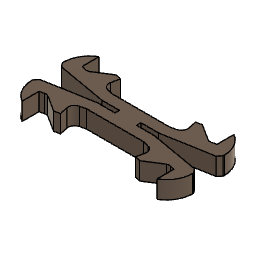
Track_Coupler (Autodesk Fusion 360 design; units mm, degrees)
Autodesk Fusion 360 part; units mm, degrees
sketch "Sketch1" plane through (0, 0, 0) normal (0, 0, 1) x (1, 0, 0)
  line L0 (-5, 0.3394) -> (-1.667, 0.3394)
  line L1 (-8, 2.6415) -> (-8, 4.0495)
  line L2 (-5, 4.2995) -> (-8, 4.2995)
  line L3 (-13, -3.75) -> (-13, -5.9)
  line L4 (-5, 3.75) -> (-13, -3.75) construction
  line L5 (11, -5.9) -> (11, -3.75)
  line L6 (-13, -3.75) -> (-21.1942, -3.75) construction
  line L7 (-5, -0.3394) -> (-11, -0.3394)
  line L8 (5, 0.3394) -> (2.3, 0.3394)
  line L9 (-13, 3.75) -> (-13, 5.9)
  line L10 (11, 5.9) -> (11, 3.3066)
  line L11 (-8, -5.75) -> (-8, -4.05)
  line L12 (-11, 5.9) -> (-11, 3.75)
  line L13 (-1.667, 0.3394) -> (-1.667, -0.3394)
  line L14 (-5, -4.05) -> (-5, -4.3)
  line L15 (13, -3.75) -> (5, -3.75)
  line L16 (13, 1.75) -> (5, 0.3394)
  line L17 (-13, -3.75) -> (-13, -1.75)
  line L18 (-1.667, -0.3394) -> (-5, -0.3394)
  line L19 (-13, -3.75) -> (-13, 3.75)
  line L20 (-13, 5.9) -> (-11, 5.9)
  line L21 (-13, -1.75) -> (-5, -0.3394)
  line L22 (-13, -3.75) -> (-5, -1.9764)
  line L23 (13, 3.75) -> (13, 5.9)
  line L24 (11, -3.75) -> (11, -3.3066)
  line L25 (-8, -4.3) -> (-8, -4.05)
  line L26 (13, -3.75) -> (5, -1.9764)
  line L27 (-13, 3.75) -> (-21.1942, 3.75) construction
  line L28 (13, 3.75) -> (5, 1.9764)
  line L29 (-11, -5.9) -> (-11, -3.3066)
  line L30 (13, -3.75) -> (13, -5.9)
  line L31 (-8, 4.0495) -> (-5, 4.0495)
  line L32 (-8, -4.05) -> (-8, -2.6415)
  line L33 (13, -3.75) -> (5, 3.75) construction
  line L34 (13, 3.75) -> (21.1942, 3.75) construction
  line L35 (-5, -4.05) -> (-5, -1.9764)
  line L36 (-11, 3.75) -> (-11, 3.3066)
  line L37 (13, 3.75) -> (13, -3.75)
  line L38 (-13, 3.75) -> (-5, -3.75) construction
  line L39 (-5, -0.3394) -> (-5, 0.3394)
  line L40 (-8, 4.2995) -> (-8, 4.0495)
  line L41 (13, -3.75) -> (13, -1.75)
  line L42 (-13, 3.75) -> (-13, 1.75)
  line L43 (13, 5.9) -> (11, 5.9)
  line L44 (-5, 1.9764) -> (-5, -1.9764)
  line L45 (-8, -4.05) -> (-5, -4.05)
  line L46 (5, -0.3394) -> (2.3, -0.3394)
  line L47 (-13, 3.75) -> (-5, 3.75)
  line L48 (5, 3.75) -> (13, 3.75)
  line L49 (-5, -4.3) -> (-8, -4.3)
  line L50 (2.3, 0.3394) -> (2.3, -0.3394)
  line L51 (-8, -4.05) -> (-5, -4.05)
  line L52 (13, -1.75) -> (5, -0.3394)
  line L53 (5, -3.75) -> (5, 3.75)
  line L54 (-13, 3.75) -> (-5, 1.9764)
  line L55 (13, 3.75) -> (13, 1.75)
  line L56 (13, 1.75) -> (21.1234, 1.75) construction
  line L57 (13, -5.9) -> (11, -5.9)
  line L58 (-13, -5.9) -> (-11, -5.9)
  line L59 (5, -3.75) -> (13, 3.75) construction
  line L60 (-8, 4.0495) -> (-5, 4.0495)
  line L61 (-5, -3.75) -> (-13, -3.75)
  line L62 (5, -1.9764) -> (5, 1.9764)
  line L63 (-13, 1.75) -> (-5, 0.3394)
  line L64 (-5, 4.0495) -> (-5, 1.9764)
  line L65 (-13, -1.75) -> (-21.1234, -1.75) construction
  line L66 (13, -3.75) -> (21.1942, -3.75) construction
  line L67 (-5, 4.0495) -> (-5, 4.2995)
  line L68 (0, -1.9764) -> (0, 1.9764)
  line L69 (5, 1.9764) -> (1.3, 1.9764)
  line L70 (0, 1.9764) -> (-5, 1.9764)
  line L71 (-5, -1.9764) -> (0, -1.9764)
  line L72 (1.3, -1.9764) -> (5, -1.9764)
  line L73 (1.3, 1.9764) -> (1.3, -1.9764)
  line L74 (-1.667, 0.3394) -> (-2.3, 0.3394)
  line L75 (-2.3, -0.3394) -> (-2.3, 0.3394)
  line L76 (-8, 4.2995) -> (-9.4644, 4.6242)
  line L77 (-9.4644, 4.6242) -> (-9.8148, 3.0439)
  line L78 (-8, 4.2995) -> (-5, 3.6344)
  line L79 (-9.4644, 4.6242) -> (-6.5356, 3.9749)
  line L80 (-6.5356, 3.9749) -> (-6.8859, 2.3945)
  line L81 (-9.4644, 4.6242) -> (-9.3238, 5.2588)
  line L82 (-6.5356, 3.9749) -> (-6.3949, 4.6095)
  line L83 (-9.3238, 5.2588) -> (-6.3949, 4.6095)
  point P0 (9, 0)
  point P1 (9, 0)
  point P2 (-9, 0)
  point P3 (-9, 0)
  dimension "d1" = 8
  dimension "d2" = 7.5
  dimension "d3" = 167.5
  dimension "d4" = 167.5
  dimension "d5" = 2
  dimension "d6" = 2
  dimension "d7" = 10
  dimension "d8" = 170
  dimension "d9" = 160
  dimension "d10" = 2.15
  dimension "d11" = 2
  dimension "d12" = 2.15
  dimension "d13" = 2
  dimension "d14" = 2.7
  dimension "d15" = 2.7
  dimension "d16" = 8
  dimension "d17" = 7.5
  dimension "d18" = 167.5
  dimension "d19" = 167.5
  dimension "d20" = 2
  dimension "d21" = 2
  dimension "d22" = 170
  dimension "d23" = 160
  dimension "d24" = 2.15
  dimension "d25" = 2
  dimension "d26" = 2.15
  dimension "d27" = 2
  dimension "d28" = 3.333
  dimension "d29" = 1.7
  dimension "d30" = 1.408
  dimension "d31" = 0.25
  dimension "d32" = 0.25
  dimension "d40" = 0.633
  dimension "d48" = 1.5
  dimension "d49" = 3
  dimension "d50" = 0.65
  dimension "d51" = 0.65
  constraint horizontal L15
  constraint perpendicular L15 L53
  constraint parallel L15 L48
  constraint parallel L37 L53
  constraint coincident P1 L33
  constraint coincident P1 L59
  constraint coincident P1 P0
  constraint horizontal L34
  constraint coincident L28.end L53
  constraint horizontal L66
  constraint coincident L26.end L53
  constraint perpendicular L48 L55
  constraint perpendicular L41 L66
  constraint horizontal L69
  constraint vertical L44
  constraint horizontal L71
  constraint vertical L62
  constraint horizontal L56
  constraint coincident L8.start L53
  constraint coincident L46.start L62
  constraint perpendicular L23 L48
  constraint perpendicular L23 L43
  constraint coincident L10.end L28
  constraint perpendicular L10 L43
  constraint perpendicular L15 L30
  constraint perpendicular L30 L57
  constraint coincident L5.end L15
  constraint perpendicular L5 L15
  constraint coincident L24.end L26
  constraint perpendicular L15 L24
  constraint perpendicular L8 L53
  constraint perpendicular L46 L53
  constraint parallel L47 L61
  constraint coincident P3 L38
  constraint coincident P3 L4
  constraint coincident P3 P2
  constraint perpendicular L17 L61
  constraint perpendicular L27 L42
  constraint perpendicular L3 L61
  constraint perpendicular L3 L58
  constraint coincident L29.end L22
  constraint perpendicular L29 L58
  constraint perpendicular L9 L47
  constraint perpendicular L9 L20
  constraint coincident L12.end L47
  constraint perpendicular L12 L47
  constraint coincident L36.end L54
  constraint perpendicular L36 L47
  constraint horizontal L0
  constraint vertical L13
  constraint horizontal L18
  constraint vertical L39
  constraint perpendicular L7 L39
  constraint perpendicular L11 L61
  constraint perpendicular L11 L51
  constraint perpendicular L35 L71
  constraint coincident L32.end L22
  constraint perpendicular L32 L51
  constraint coincident L1.start L54
  constraint perpendicular L1 L47
  constraint perpendicular L1 L31
  constraint perpendicular L31 L64
  constraint horizontal L60
  constraint vertical L67
  constraint horizontal L2
  constraint vertical L40
  constraint horizontal L45
  constraint vertical L14
  constraint horizontal L49
  constraint vertical L25
  constraint vertical L68
  constraint collinear L69 L70
  constraint coincident L68.end L69
  constraint collinear L71 L72
  constraint perpendicular L72 L73
  constraint coincident L0 L74.end
  constraint coincident L18 L75.start
  constraint perpendicular L74 L75
  constraint parallel L54 L76
  constraint coincident L54 L77.end
  constraint perpendicular L54 L77
  constraint coincident L64 L78.end
  constraint parallel L54 L78
  constraint perpendicular L77 L79
  constraint coincident L54 L80.end
  constraint perpendicular L54 L80
  constraint perpendicular L79 L81
  constraint perpendicular L79 L82
  measures "d1" distance of L33.end L23.start
  measures "d2" distance of L33.end L15.end
  measures "d3" angle of L28 L34
  measures "d4" angle of L26 L66
  measures "d5" distance of L23.start L16.start
  measures "d6" distance of L15.start L41.end
  measures "d7" distance of L28.end L44.start
  measures "d8" angle of L16 L56
  measures "d9" angle of L16 L52
  measures "d10" distance of L23.start L23.end
  measures "d11" distance of L10.start L23.end
  measures "d12" distance of L15.start L30.end
  measures "d13" distance of L30.end L5.start
  measures "d14" distance of L8.start L8.end
  measures "d15" distance of L46.start L46.end
  measures "d16" distance of L38.end L3.start
  measures "d17" distance of L4.start L38.end
  measures "d18" angle of L6 L22
  measures "d19" angle of L27 L54
  measures "d20" distance of L3.start L17.end
  measures "d21" distance of L9.start L42.end
  measures "d22" angle of L21 L65
  measures "d23" angle of L21 L63
  measures "d24" distance of L3.start L3.end
  measures "d25" distance of L29.start L3.end
  measures "d26" distance of L9.end L9.start
  measures "d27" distance of L9.end L12.start
  measures "d28" distance of L0.end L0.start
  measures "d29" distance of L11.start L11.end
  measures "d30" distance of L1.end L1.start
  measures "d31" distance of L1.end L2.end
  measures "d32" distance of L14.start L14.end
  measures "d40" distance of L0.end L74.end
  measures "d48" distance of L2.end L76.end
  measures "d49" distance of L76.end L79.end
  measures "d50" distance of L76.end L81.end
  measures "d51" distance of L79.end L82.end
extrude "Extrude1" add sketch "Sketch1" along normal blind 2.7 contours L0 L13 L18 L44 L68 L70 L71 L74 | L19 L42 L44 L54 L63 | L0 L13 L18 L74 L75 | L17 L19 L21 L22 L44 | L9 L12 L20 L47 | L36 L47 L54 | L3 L29 L58 L61 | L22 L29 L61 | L5 L15 L30 L57 | L15 L24 L26 | L26 L37 L41 L52 L53 L62 | L8 L46 L50 L53 L62 L69 L72 L73 | L16 L28 L37 L53 L55 L62 | L10 L23 L43 L48 | L10 L28 L48 makes body 1 at (9.6667, -1.7987, 2.7) makes body 2 at (-0.7667, -0.1131, 0)
move_body "Move1" bodies 1 to x (1, 0, 0) y (0, 1, 0) z (0, 0, 1) at (-1.3, 0, 0)
combine "Combine1" operation add target body 1 tool bodies 2
fillet "Fillet1" radius 4 4 edges at (11.7, 5.9, 1.35) (11.7, -5.9, 1.35) (-13, -5.9, 1.35) (-13, 5.9, 1.35) on bodies 1
chamfer "Chamfer1" distance 0.5 angle 45 4 edges at (11.7, -1.75, 1.35) (11.7, 1.75, 1.35) (-13, -1.75, 1.35) (-13, 1.75, 1.35) on bodies 1
extrude "Extrude2" add sketch "Sketch1" along normal blind 2.7 contours L1 L47 L54 L80 | L1 L47 L54 L77 | L1 L31 L47 L60 L78 L79 L80 | L1 L40 L47 L76 L77 L79 | L31 L60 L78 L79 L82 | L31 L40 L60 L78 L79 | L2 L31 L60 L78 L79 L82 | L2 L76 L79 L81 L82 L83 bodies 1
mirror "Mirror2" about plane through (0, 0, 0) normal (0, 1, 0) of "Extrude2"
ref_plane "WorkPlane1" through (-0.65, 0, 1.35) normal (1, 0, 0) x (0, 1, 0)
mirror "Mirror1" about plane through (-0.65, 0, 1.35) normal (1, 0, 0) of "Extrude2", "Mirror2"
chamfer "Chamfer2" distance 2.118 angle 45 4 edges at (-9.3238, -5.2588, 1.35) (-9.3238, 5.2588, 1.35) (8.0238, 5.2588, 1.35) (8.0238, -5.2588, 1.35) on bodies 1
move_body "Move2" bodies 1 to x (1, 0, 0) y (0, 1, 0) z (0, 0, 1) at (0.6, 0, 0)
fillet "Fillet2" radius 1 8 edges at (6.1859, 2.3945, 1.35) (6.1859, -2.3945, 1.35) (-6.2859, -2.3945, 1.35) (-6.2859, 2.3945, 1.35) (-9.2148, -3.0439, 1.35) (-9.2148, 3.0439, 1.35) (9.1148, 3.0439, 1.35) (9.1148, -3.0439, 1.35) on bodies 1
equation "d51 = d50"
named bodies: "Body2"
